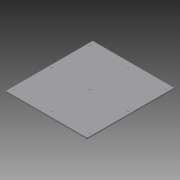
# Autodesk Inventor part: caddy2
Saved by Autodesk Inventor 2013 (Build 170138000, 138)
## iProperties
Created: 2013-11-17
Part Number: caddy2
Material: Generic
Document SubType Name: Modeling
Designer: Masta
Density: 1 g/cm^3
Author: Masta
Autodesk Inventor part; units mm, degrees
ref_plane "YZ Plane" through (0, 0, 0) normal (1, 0, 0) x (0, 1, 0)
ref_plane "XZ Plane" through (0, 0, 0) normal (0, 1, 0) x (-1, 0, 0)
ref_plane "XY Plane" through (0, 0, 0) normal (0, 0, 1) x (1, 0, 0)
sketch "Sketch1" plane through (0, 0, 0) normal (0, 0, 1) x (1, 0, 0)
  line L0 (150, 160) -> (-150, 160)
  line L1 (-150, 160) -> (-150, -160)
  line L2 (-150, -160) -> (150, -160)
  line L3 (150, -160) -> (150, 160)
  line L4 (150, 160) -> (-150, -160) construction
  line L5 (-150, 160) -> (150, -160) construction
  point P0 (0, 0)
  point P1 (0, 0)
  dimension "d0" = 300
  dimension "d1" = 320
  constraints: 12 end point, 2 midpoint, 2 parallel, 1 coincident, 1 horizontal, 1 perpendicular
  measures "d0" distance of L2.end L1.end
  measures "d1" distance of L1.end L0.end
extrude "Extrusion1" add sketch "Sketch1" against normal blind 4
hole "Hole1" at (0, 0, 0) direction (0, 0, -1) diameter 3.6 end through all
chamfer "Chamfer1" distance 2 angle 45 4 edges at (150, 160, -2) (150, -160, -2) (-150, 160, -2) (-150, -160, -2)
pattern_linear "Rectangular Pattern1" count 3 spacing 140 along (1, 0, 0) count 3 spacing 140 along (0, 1, 0) of "Hole1" first direction both ways yes second direction both ways yes
body "Solid1"
